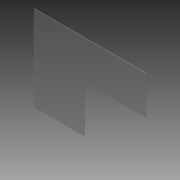
# Autodesk Inventor part: pneumatics board 1
Saved by Autodesk Inventor 2014 (Build 180170000, 170)
## iProperties
Created: 2014-01-20
Part Number: pneumatics board 1
Material: Polycarbonate, Clear
Document SubType Name: Modeling
Designer: Arpan
Density: 1.2 g/cm^3
Appearance: Polycarbonate - Clear
Author: Arpan
Autodesk Inventor part; units mm, degrees
ref_plane "YZ Plane" through (0, 0, 0) normal (1, 0, 0) x (0, 1, 0)
ref_plane "XZ Plane" through (0, 0, 0) normal (0, 1, 0) x (-1, 0, 0)
ref_plane "XY Plane" through (0, 0, 0) normal (0, 0, 1) x (1, 0, 0)
sketch "Sketch1" plane through (0, 0, 0) normal (0, 0, 1) x (1, 0, 0)
  line L0 (0, 0) -> (-150.114, 0)
  line L1 (0, 139.7) -> (0, 0)
  line L2 (184.15, 254) -> (184.15, 139.7)
  line L3 (184.15, 139.7) -> (0, 139.7)
  line L4 (184.15, 254) -> (184.15, 425.45)
  line L5 (0, 425.45) -> (0, 660.4)
  line L6 (0, 660.4) -> (-150.114, 660.4)
  line L7 (-150.114, 660.4) -> (-150.114, 0)
  line L8 (-131.064, 406.4) -> (78.486, 406.4)
  line L9 (78.486, 406.4) -> (78.486, 241.3)
  line L10 (78.486, 241.3) -> (-131.064, 241.3)
  line L11 (-131.064, 241.3) -> (-131.064, 406.4)
  line L12 (184.15, 425.45) -> (184.15, 463.55)
  line L13 (184.15, 463.55) -> (114.3, 463.55)
  line L14 (114.3, 463.55) -> (114.3, 425.45)
  line L15 (114.3, 425.45) -> (0, 425.45)
  dimension "d8" = 150.114
  dimension "d9" = 171.45
  dimension "d11" = 234.95
  dimension "d12" = 184.15
  dimension "d13" = 114.3
  dimension "d14" = 150.114
  dimension "d15" = 139.7
  dimension "d20" = 165.1
  dimension "d21" = 101.6
  dimension "d22" = 209.55
  dimension "d23" = 19.05
  dimension "d24" = 38.1
  dimension "d25" = 69.85
  dimension "d26" = 114.3
  dimension "d27" = 38.1
  constraints: 32 end point, 6 perpendicular, 4 parallel, 2 horizontal, 1 point on line
  measures "d8" distance of L0.start L0.end
  measures "d9" distance of L2.start L4.end
  measures "d11" distance of L5.start L5.end
  measures "d12" distance of L2.end L1.start
  measures "d13" distance of L2.start L2.end
  measures "d14" distance of L6.end L5.end
  measures "d15" distance between parallel lines of L0 L3
  measures "d20" distance between parallel lines of L10 L8
  measures "d21" distance between parallel lines of L3 L10
  measures "d22" distance between parallel lines of L11 L9
  measures "d23" distance between parallel lines of L7 L11
  measures "d24" distance of L4.end L12.end
  measures "d25" distance of L12.end L13.end
  measures "d26" distance between parallel lines of L5 L14
  measures "d27" distance of L13.end L14.end
extrude "Extrusion1" add sketch "Sketch1" along normal blind 1.5875
body "Solid1"
